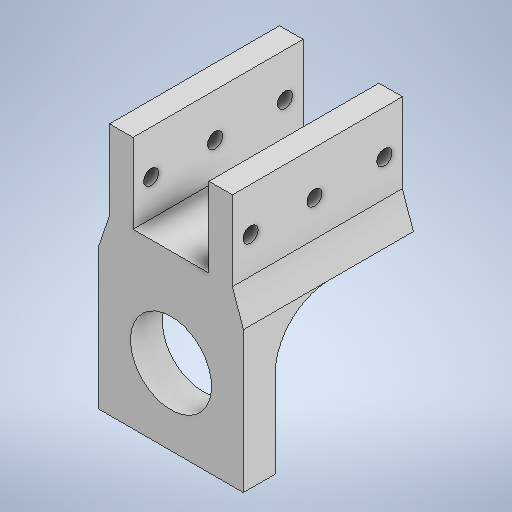
# Autodesk Inventor part: CH-4_DiffBarSupport
Saved by Autodesk Inventor 2025.1 (Build 291241020, 241B)
## iProperties
Created: 2024-12-05
Part Number: CH-4_DiffBarSupport
Material: Generic
Document SubType Name: Modeling
Designer: aidan
Density: 1 g/cm^3
Appearance: Default
Author: aidan
Autodesk Inventor part; units mm, degrees
ref_plane "YZ Plane" through (0, 0, 0) normal (1, 0, 0) x (0, 1, 0)
ref_plane "XZ Plane" through (0, 0, 0) normal (0, 1, 0) x (-1, 0, 0)
ref_plane "XY Plane" through (0, 0, 0) normal (0, 0, 1) x (1, 0, 0)
sketch "Sketch1" plane through (0, 0, 0) normal (0, 0, 1) x (1, 0, 0)
  line L0 (-25.4, -35.56) -> (25.4, -35.56)
  line L1 (25.4, -35.56) -> (25.4, 13.97)
  line L2 (25.4, 13.97) -> (-25.4, 13.97)
  line L3 (-25.4, 13.97) -> (-25.4, -35.56)
  line L4 (-25.4, -35.56) -> (25.4, 13.97) construction
  line L5 (25.4, -35.56) -> (-25.4, 13.97) construction
  line L6 (0, 25.146) -> (-12.7, 25.146)
  line L7 (-12.7, 25.146) -> (12.7, 25.146)
  line L8 (-12.7, 25.146) -> (-25.4, 13.97)
  line L9 (12.7, 25.146) -> (25.4, 13.97)
  line L10 (-12.7, 25.146) -> (-21.59, 25.146)
  line L11 (-21.59, 25.146) -> (-21.59, 50.546)
  line L12 (-21.59, 50.546) -> (-12.7, 50.546)
  line L13 (-12.7, 50.546) -> (-12.7, 25.146)
  line L14 (-21.59, 25.146) -> (-25.4, 13.97)
  line L15 (12.7, 25.146) -> (12.7, 50.546)
  line L16 (12.7, 50.546) -> (21.59, 50.546)
  line L17 (21.59, 50.546) -> (21.59, 25.146)
  line L18 (21.59, 25.146) -> (25.4, 13.97)
  line L19 (12.7, 25.146) -> (21.59, 25.146)
  circle A0 centre (0, -8.89) radius 14.224
  point P0 (0, 0)
  dimension "d1" = 49.53
  dimension "d2" = 50.8
  dimension "d6" = 8.89
  dimension "d7" = 25.4
  dimension "d8" = 8.89
  dimension "d47" = 11.176
  dimension "d51" = 28.448
  dimension "d52" = 34.036
  dimension "d53" = 43.18
  constraints: 40 end point, 6 perpendicular, 3 horizontal, 3 parallel, 3 point on line, 1 centre point
  measures "d1" distance of L0.end L1.end
  measures "d2" distance of L1.end L2.end
  measures "d6" distance of L6.end L10.end
  measures "d7" distance of L10.end L11.end
  measures "d8" distance of L15.end L16.end
  measures "d47" distance between parallel lines of L6 L2
  measures "d51" diameter of A0
  measures "d52" distance of L6.start A0.centre
  measures "d53" distance of L17.end L10.end
extrude "Extrusion1" add sketch "Sketch1" along normal blind 8.89
sketch "Sketch3" plane through (0, 0, 0) normal (0, 0, -1) x (-1, 0, 0)
  circle A0 centre (0, 0) radius 14.224
  line L0 (21.5903, 3.302) -> (-21.59, 3.302)
  line L1 (-21.59, 3.302) -> (-21.59, 25.146)
  line L2 (-21.59, 25.146) -> (21.5903, 25.146)
  line L3 (21.5903, 25.146) -> (21.5903, 3.302)
  circle A1 centre (0, 0) radius 14.224 projected
  line L4 (21.5903, 3.302) -> (-21.59, 25.146) construction
  line L5 (-21.59, 3.302) -> (21.5903, 25.146) construction
  line L6 (-25.4, -35.56) -> (-25.4, 13.97) projected
  line L7 (25.4, 13.97) -> (25.4, -35.56) projected
  line L8 (25.4, -35.56) -> (-25.4, -35.56) projected
  line L9 (25.4, 13.97) -> (25.4, -35.56) projected
  line L10 (21.59, 25.146) -> (25.4, 13.97) projected
  line L11 (21.59, 50.546) -> (21.59, 25.146) projected
  line L12 (12.7, 50.546) -> (21.59, 50.546) projected
  line L13 (12.7, 25.146) -> (12.7, 50.546) projected
  line L14 (-12.7, 25.146) -> (12.7, 25.146) projected
  line L15 (-12.7, 50.546) -> (-12.7, 25.146) projected
  line L16 (-21.59, 50.546) -> (-12.7, 50.546) projected
  line L17 (-21.59, 25.146) -> (-21.59, 50.546) projected
  line L18 (-25.4, 13.97) -> (-21.59, 25.146) projected
  line L19 (-25.4, -35.56) -> (-25.4, 13.97) projected
  line L20 (25.4, 3.302) -> (21.5903, 3.302)
  line L21 (-25.4, 3.302) -> (-21.59, 3.302)
  line L22 (0, 14.224) -> (-25.4, 14.224)
  point P0 (0.0002, 14.224)
  point P1 (-25.4, 13.97)
  point P2 (-13.8354, 3.302)
  point P3 (13.8354, 3.302)
  dimension "d13" = 28.448
  constraints: 18 end point, 3 perpendicular, 3 point on line, 2 horizontal, 2 midpoint, 2 parallel, 1 coincident, 5 other
extrude "Extrusion3" add sketch "Sketch3" along normal blind 50.8 contours A0 L22 L1 L2 L3 L0 | L0 L1 L22 A0 | L3 L10 L7 L20 | L21 L6 L18 L22 L1 | L22 L18 L1 | L2 L13 L12 L11 | L17 L16 L15 L2
sketch "Sketch5" plane through (21.59, 50.546, 8.89) normal (1, 0, 0) x (0, 0, -1)
  line L0 (59.69, -25.4) -> (59.69, 0) projected
  line L1 (0, -23.5788) -> (57.5469, -23.5788) projected
  line L2 (57.5469, 0) -> (57.5469, -23.5788)
  line L3 (59.69, 0) -> (59.69, -25.4) projected
  line L4 (59.69, 0) -> (0, 0) projected
  line L5 (0, -25.4) -> (0, 0) projected
  line L6 (59.69, -25.4) -> (0, -25.4) projected
  line L7 (0, -25.4) -> (0, -12.7)
  line L8 (0, -12.7) -> (57.5469, -12.7)
  circle A0 centre (6.35, -12.7) radius 2.6543
  circle A1 centre (53.34, -12.7) radius 2.6543
  circle A2 centre (28.7734, -12.7) radius 2.6543
  point P0 (8.89, -50.546)
  point P1 (59.69, -25.4)
  point P2 (31.4277, -12.7)
  point P3 (26.1191, -12.7)
  point P4 (55.9943, -12.7)
  point P5 (50.6857, -12.7)
  point P6 (9.0043, -12.7)
  point P7 (3.6957, -12.7)
  dimension "d39" = 12.7
  dimension "d40" = 5.3086
  dimension "d41" = 6.35
  dimension "d42" = 5.3086
  dimension "d43" = 6.35
  dimension "d44" = 5.3086
  dimension "d46" = 0
  constraints: 4 end point, 3 centre point, 2 midpoint, 2 point on line, 1 horizontal, 4 other
  measures "d39" distance of L5.start L7.end
  measures "d40" diameter of A0
  measures "d41" distance from line of L5 A0.centre
  measures "d42" diameter of A1
  measures "d44" diameter of A2
  measures "d46" angle of L6 L8
extrude "Extrusion4" cut sketch "Sketch5" against normal up to surface (43.18 mm away) contours A1 L8 | L8 A1 | A0 L8 | L8 A0 | A2 L8 | L8 A2
sketch "Sketch9" plane through (0, 0, -50.8) normal (0, 0, -1) x (-1, 0, 0)
  line L0 (-21.59, 50.546) -> (-12.7, 50.546) projected
  line L1 (13.335, -0.254) -> (-13.335, -0.254)
  line L2 (-13.335, -0.254) -> (-13.335, 50.546)
  line L3 (-13.335, 50.546) -> (13.335, 50.546)
  line L4 (13.335, 50.546) -> (13.335, -0.254)
  line L5 (-12.7, 25.146) -> (12.7, 25.146) projected
  line L6 (13.335, -0.254) -> (-13.335, 50.546) construction
  line L7 (-13.335, -0.254) -> (13.335, 50.546) construction
  line L8 (-25.4, -35.56) -> (-25.4, 13.97) projected
  line L9 (25.4, -13.97) -> (-25.4, -13.97)
  line L10 (-25.4, -13.97) -> (-25.4, 13.97)
  line L11 (-25.4, 13.97) -> (25.4, 13.97)
  line L12 (25.4, 13.97) -> (25.4, -13.97)
  line L13 (25.4, -13.97) -> (-25.4, 13.97) construction
  line L14 (-25.4, -13.97) -> (25.4, 13.97) construction
  point P0 (0, 0)
  point P1 (0, 25.146)
  point P2 (-13.335, 13.97)
  point P3 (13.335, 13.97)
  point P4 (-12.7, 50.546)
  dimension "d27" = 26.67
  constraints: 24 end point, 5 midpoint, 4 parallel, 2 horizontal, 2 perpendicular, 1 point on line
  measures "d27" distance of L2.end L3.end
extrude "Extrusion5" cut sketch "Sketch9" against normal blind 42.8625
sketch "Sketch11" plane through (0, 0, 0) normal (0, 0, -1) x (-1, 0, 0)
  line L0 (25.4, 3.302) -> (13.8354, 3.302) projected
  line L1 (-13.8354, 3.302) -> (-25.4, 3.302) projected
  line L2 (-25.4, -35.56) -> (-25.4, 3.302) projected
  line L3 (25.4, -35.56) -> (-25.4, -35.56) projected
  line L4 (25.4, 3.302) -> (25.4, -35.56) projected
  line L5 (12.7, 25.146) -> (12.7, 50.546) projected
  line L6 (-12.7, 25.146) -> (12.7, 25.146) projected
  line L7 (-12.7, 50.546) -> (-12.7, 25.146) projected
  line L8 (-13.335, 50.546) -> (-12.7, 50.546) projected
  line L9 (-13.335, 13.97) -> (-13.335, 50.546) projected
  line L10 (-25.4, 13.97) -> (-13.335, 13.97) projected
  line L11 (-25.4, 3.302) -> (-25.4, 13.97) projected
  line L12 (-13.8354, 3.302) -> (-25.4, 3.302) projected
  arc A0 (13.8354, 3.302) -> (-13.8354, 3.302) centre (0, 0) ccw projected
  line L13 (25.4, 3.302) -> (13.8354, 3.302) projected
  line L14 (25.4, 13.97) -> (25.4, 3.302) projected
  line L15 (13.335, 13.97) -> (25.4, 13.97) projected
  line L16 (13.335, 50.546) -> (13.335, 13.97) projected
  line L17 (12.7, 50.546) -> (13.335, 50.546) projected
  arc A1 (13.8354, 3.302) -> (-13.8354, 3.302) centre (0, 0) ccw projected
extrude "Extrusion6" add sketch "Sketch11" along normal blind 2.286 contours L4 L3 L2 L1 A0 L0
sketch "Sketch12" plane through (0, 0, -7.9375) normal (0, 0, -1) x (-1, 0, 0)
  line L0 (12.7, 25.146) -> (12.7, 50.546) projected
  line L1 (-12.7, 25.146) -> (12.7, 25.146) projected
  line L2 (-12.7, 50.546) -> (-12.7, 25.146) projected
  line L3 (-13.335, 50.546) -> (-12.7, 50.546) projected
  line L4 (-13.335, 13.97) -> (-13.335, 50.546) projected
  line L5 (-25.4, 13.97) -> (-13.335, 13.97) projected
  line L6 (-25.4, 3.302) -> (-25.4, 13.97) projected
  line L7 (-13.8354, 3.302) -> (-25.4, 3.302) projected
  arc A0 (13.8354, 3.302) -> (-13.8354, 3.302) centre (0, 0) ccw projected
  line L8 (25.4, 3.302) -> (13.8354, 3.302) projected
  line L9 (25.4, 13.97) -> (25.4, 3.302) projected
  line L10 (13.335, 13.97) -> (25.4, 13.97) projected
  line L11 (13.335, 50.546) -> (13.335, 13.97) projected
  line L12 (12.7, 50.546) -> (13.335, 50.546) projected
extrude "Extrusion7" cut sketch "Sketch12" against normal blind 5.6515
sketch "Sketch13" plane through (0, 0, -2.286) normal (0, 0, -1) x (-1, 0, 0)
  line L0 (-12.7, 25.146) -> (12.7, 25.146) projected
  line L1 (-13.335, 13.97) -> (-13.335, 50.546) projected
  line L2 (12.7, 25.146) -> (-13.335, 25.146)
  line L3 (-13.335, 25.146) -> (-13.335, 50.546)
  line L4 (-13.335, 50.546) -> (12.7, 50.546)
  line L5 (12.7, 50.546) -> (12.7, 25.146)
  line L6 (13.335, 50.546) -> (13.335, 13.97) projected
  line L7 (12.7, 50.546) -> (13.335, 50.546)
  line L8 (13.335, 50.546) -> (13.335, 25.146)
  line L9 (13.335, 25.146) -> (12.7, 25.146)
  line L10 (12.7, 25.146) -> (12.7, 50.546)
  point P0 (0, 0)
  point P1 (-13.335, 25.146)
  constraints: 16 end point, 4 parallel, 2 horizontal, 2 perpendicular, 2 point on line
extrude "Extrusion8" cut sketch "Sketch13" against normal blind 37.211
sketch "Sketch14" plane through (0, 0, -2.286) normal (0, 0, -1) x (-1, 0, 0)
  circle A0 centre (0, 0) radius 14.224 projected
  line L0 (25.4, 13.97) -> (25.4, -35.56) projected
  line L1 (13.335, 25.146) -> (-13.335, 25.146) projected
  line L2 (-13.335, 13.97) -> (-13.335, 25.146) projected
  line L3 (-25.4, 13.97) -> (-13.335, 13.97) projected
  line L4 (-25.4, -35.56) -> (-25.4, 13.97) projected
  line L5 (-25.4, -35.56) -> (25.4, -35.56) projected
  line L6 (25.4, 13.97) -> (25.4, -35.56) projected
  line L7 (13.335, 13.97) -> (25.4, 13.97) projected
  line L8 (13.335, 25.146) -> (13.335, 13.97) projected
  line L9 (-13.335, 13.97) -> (-13.335, 50.546) projected
  line L10 (-13.335, 50.546) -> (-21.59, 50.546) projected
  line L11 (-21.59, 50.546) -> (-21.59, 25.146) projected
  line L12 (-21.59, 25.146) -> (-25.4, 13.97) projected
  line L13 (-25.4, 13.97) -> (-13.335, 13.97) projected
  line L14 (13.335, 50.546) -> (13.335, 13.97) projected
  line L15 (13.335, 13.97) -> (25.4, 13.97) projected
  line L16 (25.4, 13.97) -> (21.59, 25.146) projected
  line L17 (21.59, 25.146) -> (21.59, 50.546) projected
  line L18 (21.59, 50.546) -> (13.335, 50.546) projected
  line L19 (-21.59, 25.146) -> (21.59, 25.146)
  line L20 (-25.4, 15.2659) -> (25.4, 15.2659)
  point P0 (25.4, 14.224)
  point P1 (25.4, 13.97)
  point P2 (-25.4, 13.97)
  point P3 (25.4, 13.97)
  point P4 (24.9582, 15.2659)
  point P5 (13.335, 15.2659)
  point P6 (-13.335, 15.2659)
  point P7 (-24.9582, 15.2659)
  constraints: 4 end point, 3 point on line, 1 horizontal, 1 perpendicular
extrude "Extrusion9" add sketch "Sketch14" along normal up to surface (48.514 mm away) contours L20 L8 L19 L16 | L20 L2 L1 L8 | L20 L12 L19 L2
sketch "Sketch15" plane through (0, -8.89, 0) normal (0, 0, 1) x (1, 0, 0)
  circle A0 centre (0, 0) radius 14.224 projected
  point P0 (0, 8.89)
extrude "Extrusion10" cut sketch "Sketch15" against normal blind 33.9725
sketch "Sketch16" plane through (-21.59, 50.546, 8.89) normal (0, 1, 0) x (1, 0, 0)
  line L0 (8.255, 0) -> (8.255, 59.69) projected
  line L1 (0, 59.69) -> (8.255, 59.69) projected
  line L2 (0, 59.69) -> (0, 0) projected
  line L3 (8.255, 0) -> (0, 0) projected
  line L4 (34.925, 59.69) -> (34.925, 0) projected
  line L5 (43.18, 0) -> (34.925, 0) projected
  line L6 (43.18, 59.69) -> (43.18, 0) projected
  line L7 (34.925, 59.69) -> (43.18, 59.69) projected
  point P0 (21.59, 8.89)
extrude "Extrusion11" add sketch "Sketch16" along normal blind 2.54
sketch "Sketch17" plane through (0, 0, -2.286) normal (0, 0, -1) x (-1, 0, 0)
  line L0 (-25.4, 13.97) -> (-13.335, 13.97) projected
  line L1 (13.335, 15.2659) -> (13.335, 13.97) projected
  line L2 (-13.335, 13.97) -> (13.335, 13.97)
  line L3 (13.335, 13.97) -> (13.335, 15.2659)
  line L4 (13.335, 15.2659) -> (-13.335, 15.2659)
  line L5 (-13.335, 15.2659) -> (-13.335, 13.97)
  point P0 (0, 0)
  constraints: 8 end point, 2 parallel, 1 horizontal, 1 perpendicular
extrude "Extrusion12" add sketch "Sketch17" along normal up to surface (48.514 mm away)
fillet "Fillet5" radius 19.05 1 edges at (0, 13.97, -2.286)
equation "\"d9\" = d6"
body "Solid1"
